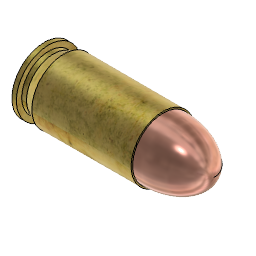
45ACP_FMJ (Autodesk Fusion 360 design; units mm, degrees)
Autodesk Fusion 360 part; units mm, degrees
sketch "スケッチ1" plane through (0, 0, 0) normal (0, 0, 1) x (1, 0, 0)
  line L0 (0, 0) -> (32.39, 0)
  line L1 (0.38, 6.095) -> (0.38, -6.095) construction
  line L2 (0, 5.5523) -> (0, -5.5523)
  line L3 (0.38, 6.095) -> (0, 5.5523)
  line L4 (0, -5.5523) -> (0.38, -6.095)
  line L5 (1.24, 5.08) -> (1.24, -5.08) construction
  line L6 (0.38, 6.095) -> (1.24, 6.095)
  line L7 (1.24, -6.095) -> (0.38, -6.095)
  line L8 (2.13, 5.08) -> (2.13, -5.08) construction
  line L9 (2.13, -5.08) -> (1.24, -5.08)
  line L10 (2.13, 5.08) -> (1.24, 5.08)
  line L11 (1.24, 6.095) -> (1.24, 5.08)
  line L12 (1.24, -5.08) -> (1.24, -6.095)
  line L13 (4.11, 6.0457) -> (4.11, -6.0443) construction
  line L14 (2.13, 5.08) -> (4.11, 6.0457)
  line L15 (22.81, 6.005) -> (22.81, -6.005)
  line L16 (4.11, 6.0457) -> (22.81, 6.005)
  line L17 (4.11, -6.0443) -> (22.81, -6.005)
  line L18 (2.13, -5.08) -> (4.11, -6.0443)
  ellipse E0 centre (22.81, 0) end of major axis (32.39, 0) minor radius 5.74
  line L19 (13.23, 0) -> (32.39, 0) construction
  line L20 (22.81, -5.74) -> (22.81, 5.74) construction
  dimension "d1" = 32.39
  dimension "d2" = 12.19
  dimension "d3" = 0.38
  dimension "d4" = 35
  dimension "d6" = 1.24
  dimension "d7" = 10.16
  dimension "d8" = 0.89
  dimension "d9" = 12.09
  dimension "d10" = 4.11
  dimension "d11" = 26
  dimension "d12" = 12.01
  dimension "d13" = 22.81
  dimension "d14" = 11.48
  constraint coincident L0.start origin
  constraint horizontal L0
  constraint perpendicular L0 L1
  constraint symmetric L0 L1.start L1.end
  constraint vertical L2
  constraint midpoint L0.start L2
  constraint perpendicular L0 L5
  constraint perpendicular L5 L6
  constraint perpendicular L5 L7
  constraint perpendicular L0 L8
  constraint perpendicular L5 L9
  constraint perpendicular L5 L10
  constraint symmetric L0 L8.start L8.end
  constraint perpendicular L0 L11
  constraint perpendicular L0 L12
  constraint vertical L13
  constraint perpendicular L0 L15
  constraint symmetric L0 L15.start L15.end
  constraint coincident E0 L19.start
  constraint coincident E0 L0.end
  constraint coincident E0 L20.start
  constraint coincident E0 L20.end
  constraint midpoint L15 E0.centre
  constraint coincident L0.end L19.end
  measures "d1" distance of L0.start L0.end
  measures "d2" distance of L1.start L1.end
  measures "d3" distance of L0.start L1
  measures "d4" angle of L1 L3
  measures "d6" distance of L2 L5
  measures "d7" distance of L8.start L8.end
  measures "d8" distance of L5 L8
  measures "d9" distance of L13.start L13.end
  measures "d10" distance of L2 L13
  measures "d11" angle of L0 L14
  measures "d12" distance of L15.start L15.end
  measures "d13" distance of L2 L15
revolve "回転1" add sketch "スケッチ1" angle 360 about axis through (0, 0, 0) along (1, 0, 0) contours L0 L2 L3 L6 L10 L11 L14 L15 L16 E0 | L0 L15 E0 picked at (16.8332, 0.9378) makes body 1
sketch "スケッチ2" plane through (22.81, 0, 0) normal (1, 0, 0) x (0, 1, 0)
  circle A0 centre (0, 0) radius 6.005
  circle A1 centre (0, 0) radius 5
  dimension "d16" = 10
  constraint concentric A0 A1
  measures "d16" diameter of A1
extrude "押し出し1" cut sketch "スケッチ2" against normal blind 6 contours A1 bodies 1
revolve "回転2" add sketch "スケッチ1" angle 360 about axis through (0, 0, 0) along (1, 0, 0) separate body contours L0 L15 E0 picked at (28.7514, 0.9746) makes body 2
sketch "スケッチ3" plane through (22.81, 0, 0) normal (-1, 0, 0) x (0, -1, 0)
  circle A0 centre (0, 0) radius 5.74
  circle A1 centre (0, 0) radius 4.8
  dimension "d20" = 9.6
  constraint concentric A0 A1
  measures "d20" diameter of A1
extrude "押し出し2" add sketch "スケッチ3" along normal blind 5 contours A1 bodies 2
sketch "スケッチ4" plane through (0, 0, 0) normal (-1, 0, 0) x (0, -1, 0)
  circle A0 centre (0, 0) radius 5.5523
  circle A1 centre (0, 0) radius 2.25
  dimension "d23" = 4.5
  constraint coincident A0.centre A1.centre
  measures "d23" diameter of A1
extrude "押し出し3" cut sketch "スケッチ4" against normal blind 1 contours A1 bodies 1
chamfer "面取り1" distance 0.3 angle 45 1 edges at (0, 2.0977, 0.8136) on bodies 1
extrude "押し出し4" add 1 faces at (1, -1.1556, -0.7479) along direction (-1, 0, 0) blind 1 on bodies 1 bodies 1
extrude "押し出し5" cut 1 faces at (16.81, 1.3101, -1.9935) along direction (-1, 0, 0) blind 10 on bodies 1 bodies 1
